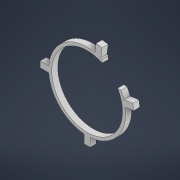
# Autodesk Inventor part: Clip_TestFitV1
Saved by Autodesk Inventor 2022 (Build 260153000, 153)
## iProperties
Created: 2023-05-05
Part Number: Clip_TestFitV1
Material: Generic
Document SubType Name: Modeling
Designer: User
Density: 1 g/cm^3
Appearance: Default
Author: User
Autodesk Inventor part; units mm, degrees
ref_plane "YZ Plane" through (0, 0, 0) normal (1, 0, 0) x (0, 1, 0)
ref_plane "XZ Plane" through (0, 0, 0) normal (0, 1, 0) x (-1, 0, 0)
ref_plane "XY Plane" through (0, 0, 0) normal (0, 0, 1) x (1, 0, 0)
sketch "Sketch1" plane through (0, 0, 0) normal (0, 0, 1) x (1, 0, 0)
  arc A0 (-25.4018, 15) -> (25.4018, 15) centre (0, 0) ccw
  line L0 (25.4018, 15) -> (28.2666, 15)
  line L1 (-39, 2.5) -> (-32, 2.5)
  line L2 (-32, -2.5) -> (-39, -2.5)
  line L3 (-39, -2.5) -> (-39, 2.5)
  line L4 (-32, 2.5) -> (-31.9022, 2.5)
  line L5 (-32, -2.5) -> (-31.9022, -2.5)
  line L6 (2.5, -32) -> (2.5, -39)
  line L7 (2.5, -39) -> (-2.5, -39)
  line L8 (-2.5, -39) -> (-2.5, -32)
  line L9 (-2.5, -32) -> (-2.5, -31.9022)
  line L10 (2.5, -32) -> (2.5, -31.9022)
  arc A1 (-28.2666, 15) -> (-31.9022, 2.5) centre (0, 0) ccw
  arc A2 (-31.9022, -2.5) -> (-2.5, -31.9022) centre (0, 0) ccw
  arc A3 (2.5, -31.9022) -> (31.9022, -2.5) centre (0, 0) ccw
  arc A4 (12.5, 26.7208) -> (25.4018, 15) centre (0, 0) ccw
  line L11 (12.5, 29.4576) -> (12.5, 26.7208)
  arc A5 (-2.5, 31.9022) -> (-31.9022, 2.5) centre (0, 0) ccw
  arc A6 (-31.9022, -2.5) -> (-2.5, -31.9022) centre (0, 0) ccw
  arc A7 (2.5, -31.9022) -> (31.9022, -2.5) centre (0, 0) ccw
  line L12 (6.5, 31.3329) -> (7.5001, 38.3601)
  line L13 (6.5, 31.3329) -> (13.598, 31.3329) construction
  line L14 (7.5001, 38.3601) -> (12.4502, 37.6556)
  line L15 (12.4502, 37.6556) -> (11.3493, 29.9198)
  arc A8 (12.5, 29.4576) -> (11.3493, 29.9198) centre (0, 0) ccw
  arc A9 (12.5, 29.4576) -> (11.3493, 29.9198) centre (0, 0) ccw
  arc A10 (6.5, 31.3329) -> (2.5, 31.9022) centre (0, 0) ccw
  arc A11 (6.5, 31.3329) -> (-31.9022, 2.5) centre (0, 0) ccw
  arc A12 (-31.9022, -2.5) -> (-2.5, -31.9022) centre (0, 0) ccw
  arc A13 (2.5, -31.9022) -> (31.9022, -2.5) centre (0, 0) ccw
  line L16 (31.682, 4.5) -> (32.601, 4.5) construction
  line L17 (31.682, 4.5) -> (39.0737, 4.5) construction
  line L18 (-2.5, 31.9022) -> (4.598, 31.9022) construction
  line L19 (31.682, 4.5) -> (38.7092, 5.5001)
  line L20 (31.682, 4.5) -> (38.78, 4.5) construction
  line L21 (38.7092, 5.5001) -> (38.0047, 10.4502)
  line L22 (38.0047, 10.4502) -> (30.5898, 9.3949)
  arc A14 (30.5898, 9.3949) -> (28.2666, 15) centre (0, 0) ccw
  arc A15 (31.9022, 2.5) -> (31.682, 4.5) centre (0, 0) ccw
  arc A16 (30.5898, 9.3949) -> (28.2666, 15) centre (0, 0) ccw
  arc A17 (31.9022, 2.5) -> (31.682, 4.5) centre (0, 0) ccw
  arc A18 (30.5898, 9.3949) -> (28.2666, 15) centre (0, 0) ccw
  arc A19 (31.9022, 2.5) -> (31.682, 4.5) centre (0, 0) ccw
  arc A20 (30.5898, 9.3949) -> (28.2666, 15) centre (0, 0) ccw
  arc A21 (12.5, 29.4576) -> (11.3493, 29.9198) centre (0, 0) ccw
  arc A22 (2.5, -31.9022) -> (31.682, 4.5) centre (0, 0) ccw
  arc A23 (6.5, 31.3329) -> (-31.9022, 2.5) centre (0, 0) ccw
  arc A24 (-31.9022, -2.5) -> (-2.5, -31.9022) centre (0, 0) ccw
  point P0 (11.5, 29.8622)
  point P1 (2.5, 31.9022)
  point P2 (31.9022, -2.5)
  dimension "d78" = 7.098
  dimension "d79" = 81.9
  dimension "d80" = 5
  dimension "d81" = 90
  dimension "d82" = 90
  dimension "d94" = 7.098
  dimension "d95" = 8.1
  dimension "d96" = 5
  dimension "d97" = 90
  dimension "d98" = 90
  constraints: 52 point on circle, 46 end point, 25 centre point, 10 coincident, 8 horizontal, 2 equal length, 2 parallel, 2 perpendicular, 2 vertical
  measures "d78" distance of L12.start L12.end
  measures "d79" angle of L13 L12
  measures "d80" distance of L12.end L14.end
  measures "d81" angle of L12 L14
  measures "d82" angle of L14 L15
  measures "d94" distance of L17.start L19.end
  measures "d95" angle of L20 L19
  measures "d96" distance of L19.end L21.end
  measures "d97" angle of L21 L19
  measures "d98" angle of L22 L21
extrude "Extrusion7" add sketch "Sketch1" along normal blind 5
body "Solid5"
